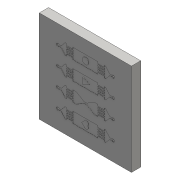
# Autodesk Inventor part: Flow-Analysis
Saved by Autodesk Inventor 2016 (Build 200138000, 138)
## iProperties
Created: 2018-10-05
Part Number: Flow-Analysis
Material: Genérico
Document SubType Name: Modeling
Designer: Joseahpacho
Density: 1 g/cm^3
Appearance: Valor por defecto
Author: Joseahpacho
Autodesk Inventor part; units mm, degrees
ref_plane "YZ Plane" through (0, 0, 0) normal (1, 0, 0) x (0, 1, 0)
ref_plane "XZ Plane" through (0, 0, 0) normal (0, 1, 0) x (-1, 0, 0)
ref_plane "XY Plane" through (0, 0, 0) normal (0, 0, 1) x (1, 0, 0)
sketch "Boceto1" plane through (0, 0, 0) normal (0, 1, 0) x (-1, 0, 0)
  line L0 (35.2407, 11.475) -> (35.2407, 10.885)
  line L1 (35.2407, 10.885) -> (31.7746, 10.885)
  line L2 (31.7746, 10.885) -> (31.7746, 11.475)
  line L3 (31.7746, 11.475) -> (35.2407, 11.475)
  line L4 (35.2407, 12.95) -> (35.2407, 12.065)
  line L5 (31.7746, 12.065) -> (31.7746, 12.95)
  line L6 (35.2407, 12.065) -> (31.7746, 12.065)
  line L7 (35.2407, 9.115) -> (35.2407, 8.525)
  line L8 (35.2407, 8.525) -> (31.7746, 8.525)
  line L9 (31.7746, 8.525) -> (31.7746, 9.115)
  line L10 (31.7746, 9.115) -> (35.2407, 9.115)
  line L11 (31.7746, 7.935) -> (35.2407, 7.935)
  line L12 (35.2407, 7.935) -> (35.2407, 7.05)
  line L13 (31.7746, 7.05) -> (31.7746, 7.935)
  line L14 (31.7746, 17.935) -> (35.2407, 17.935)
  line L15 (38.1349, 9.55) -> (36.043, 7.05)
  line L16 (35.2407, 10.295) -> (35.2407, 9.705)
  line L17 (35.2407, 9.705) -> (31.7746, 9.705)
  line L18 (31.7746, 9.705) -> (31.7746, 10.295)
  line L19 (31.7746, 10.295) -> (35.2407, 10.295)
  line L20 (31.7746, 17.05) -> (31.7746, 17.935)
  line L21 (35.2407, 17.935) -> (35.2407, 17.05)
  line L22 (35.2407, 19.115) -> (35.2407, 18.525)
  line L23 (35.2407, 18.525) -> (31.7746, 18.525)
  line L24 (31.7746, 18.525) -> (31.7746, 19.115)
  line L25 (31.7746, 19.115) -> (35.2407, 19.115)
  line L26 (18.2254, 29.705) -> (18.2254, 30.295)
  line L27 (35.2407, 31.475) -> (35.2407, 30.885)
  line L28 (38.1349, 10.45) -> (36.043, 12.95)
  line L29 (35.2407, 30.885) -> (31.7746, 30.885)
  line L30 (35.2407, 21.475) -> (35.2407, 20.885)
  line L31 (35.2407, 20.885) -> (31.7746, 20.885)
  line L32 (31.7746, 20.885) -> (31.7746, 21.475)
  line L33 (31.7746, 21.475) -> (35.2407, 21.475)
  line L34 (38.1349, 19.55) -> (36.043, 17.05)
  line L35 (31.7746, 30.885) -> (31.7746, 31.475)
  line L36 (38.1349, 20.45) -> (36.043, 22.95)
  line L37 (31.7746, 31.475) -> (35.2407, 31.475)
  line L38 (31.7746, 22.065) -> (31.7746, 22.95)
  line L39 (35.2407, 22.065) -> (31.7746, 22.065)
  line L40 (35.2407, 22.95) -> (35.2407, 22.065)
  line L41 (35.2407, 20.295) -> (35.2407, 19.705)
  line L42 (35.2407, 19.705) -> (31.7746, 19.705)
  line L43 (31.7746, 19.705) -> (31.7746, 20.295)
  line L44 (31.7746, 20.295) -> (35.2407, 20.295)
  line L45 (31.7746, 37.05) -> (31.7746, 37.935)
  line L46 (31.7746, 27.05) -> (31.7746, 27.935)
  line L47 (14.7593, 32.95) -> (14.7593, 32.065)
  line L48 (14.7593, 32.065) -> (18.2254, 32.065)
  line L49 (14.7593, 30.295) -> (14.7593, 29.705)
  line L50 (14.7593, 29.705) -> (18.2254, 29.705)
  line L51 (35.2407, 42.95) -> (35.2407, 42.065)
  line L52 (18.2254, 30.295) -> (14.7593, 30.295)
  line L53 (35.2407, 42.065) -> (31.7746, 42.065)
  line L54 (14.7593, 37.935) -> (14.7593, 37.05)
  line L55 (35.2407, 37.935) -> (35.2407, 37.05)
  line L56 (14.7593, 39.115) -> (14.7593, 38.525)
  line L57 (14.7593, 38.525) -> (18.2254, 38.525)
  line L58 (18.2254, 38.525) -> (18.2254, 39.115)
  line L59 (18.2254, 39.115) -> (14.7593, 39.115)
  line L60 (11.8651, 39.55) -> (13.957, 37.05)
  line L61 (14.7593, 40.295) -> (14.7593, 39.705)
  line L62 (14.7593, 39.705) -> (18.2254, 39.705)
  line L63 (18.2254, 39.705) -> (18.2254, 40.295)
  line L64 (18.2254, 40.295) -> (14.7593, 40.295)
  line L65 (38.1349, 29.55) -> (36.043, 27.05)
  line L66 (38.1349, 40.45) -> (36.043, 42.95)
  line L67 (11.8651, 30.45) -> (13.957, 32.95)
  line L68 (14.7593, 41.475) -> (14.7593, 40.885)
  line L69 (14.7593, 40.885) -> (18.2254, 40.885)
  line L70 (18.2254, 40.885) -> (18.2254, 41.475)
  line L71 (18.2254, 41.475) -> (14.7593, 41.475)
  line L72 (11.8651, 40.45) -> (13.957, 42.95)
  line L73 (14.7593, 42.95) -> (14.7593, 42.065)
  line L74 (18.2254, 42.065) -> (18.2254, 42.95)
  arc A0 (25.3787, 11.658) -> (23.7446, 10.0239) centre (24.5617, 10.8409) ccw
  arc A1 (23.7446, 10.0239) -> (25.3787, 8.3899) centre (24.5617, 9.2069) ccw
  line L75 (25.3787, 11.658) -> (27.0127, 10.0239)
  line L76 (27.0127, 10.0239) -> (25.3787, 8.3899)
  line L77 (25.7518, 20.4473) -> (29.9578, 22.95)
  line L78 (22.7639, 29.8706) -> (26.3406, 28.0945)
  line L79 (26.3406, 31.6467) -> (26.3406, 28.0945)
  line L80 (22.7639, 29.8706) -> (26.3406, 31.6467)
  line L81 (18.2254, 32.065) -> (18.2254, 32.95)
  line L82 (18.2254, 37.05) -> (18.2254, 37.935)
  circle A2 centre (25, 39.8706) radius 1.7363
  line L83 (18.2254, 37.935) -> (14.7593, 37.935)
  line L84 (24.2482, 20.4473) -> (25.7518, 20.4473)
  line L85 (24.2482, 20.4473) -> (20.0422, 22.95)
  line L86 (24.2482, 19.5527) -> (25.7518, 19.5527)
  line L87 (25.7518, 19.5527) -> (29.9578, 17.05)
  line L88 (24.2482, 19.5527) -> (20.0422, 17.05)
  line L89 (14.7593, 12.95) -> (14.7593, 12.065)
  line L90 (18.2254, 12.065) -> (18.2254, 12.95)
  line L91 (14.7593, 12.065) -> (18.2254, 12.065)
  line L92 (14.7593, 11.475) -> (14.7593, 10.885)
  line L93 (14.7593, 10.885) -> (18.2254, 10.885)
  line L94 (18.2254, 10.885) -> (18.2254, 11.475)
  line L95 (18.2254, 11.475) -> (14.7593, 11.475)
  line L96 (14.7593, 10.295) -> (14.7593, 9.705)
  line L97 (14.7593, 9.705) -> (18.2254, 9.705)
  line L98 (18.2254, 9.705) -> (18.2254, 10.295)
  line L99 (18.2254, 10.295) -> (14.7593, 10.295)
  line L100 (14.7593, 21.475) -> (14.7593, 20.885)
  line L101 (14.7593, 20.885) -> (18.2254, 20.885)
  line L102 (18.2254, 20.885) -> (18.2254, 21.475)
  line L103 (18.2254, 21.475) -> (14.7593, 21.475)
  line L104 (14.7593, 27.935) -> (14.7593, 27.05)
  line L105 (18.2254, 22.065) -> (18.2254, 22.95)
  line L106 (14.7593, 22.065) -> (18.2254, 22.065)
  line L107 (14.7593, 22.95) -> (14.7593, 22.065)
  line L108 (18.2254, 17.935) -> (14.7593, 17.935)
  line L109 (18.2254, 17.05) -> (18.2254, 17.935)
  line L110 (14.7593, 17.935) -> (14.7593, 17.05)
  line L111 (14.7593, 19.115) -> (14.7593, 18.525)
  line L112 (14.7593, 18.525) -> (18.2254, 18.525)
  line L113 (18.2254, 18.525) -> (18.2254, 19.115)
  line L114 (18.2254, 19.115) -> (14.7593, 19.115)
  line L115 (14.7593, 20.295) -> (14.7593, 19.705)
  line L116 (14.7593, 19.705) -> (18.2254, 19.705)
  line L117 (18.2254, 19.705) -> (18.2254, 20.295)
  line L118 (18.2254, 20.295) -> (14.7593, 20.295)
  line L119 (18.2254, 27.05) -> (18.2254, 27.935)
  line L120 (14.7593, 29.115) -> (14.7593, 28.525)
  line L121 (14.7593, 28.525) -> (18.2254, 28.525)
  line L122 (18.2254, 28.525) -> (18.2254, 29.115)
  line L123 (18.2254, 29.115) -> (14.7593, 29.115)
  line L124 (14.7593, 9.115) -> (14.7593, 8.525)
  line L125 (14.7593, 8.525) -> (18.2254, 8.525)
  line L126 (18.2254, 8.525) -> (18.2254, 9.115)
  line L127 (18.2254, 9.115) -> (14.7593, 9.115)
  line L128 (18.2254, 27.935) -> (14.7593, 27.935)
  line L129 (11.8651, 19.55) -> (13.957, 17.05)
  line L130 (11.8651, 10.45) -> (13.957, 12.95)
  line L131 (11.8651, 9.55) -> (13.957, 7.05)
  line L132 (11.8651, 29.55) -> (13.957, 27.05)
  line L133 (14.7593, 31.475) -> (14.7593, 30.885)
  line L134 (14.7593, 30.885) -> (18.2254, 30.885)
  line L135 (18.2254, 30.885) -> (18.2254, 31.475)
  line L136 (18.2254, 31.475) -> (14.7593, 31.475)
  line L137 (11.8651, 20.45) -> (13.957, 22.95)
  line L138 (31.7746, 27.935) -> (35.2407, 27.935)
  line L139 (18.2254, 7.935) -> (14.7593, 7.935)
  line L140 (14.7593, 7.935) -> (14.7593, 7.05)
  line L141 (18.2254, 7.05) -> (18.2254, 7.935)
  line L142 (35.2407, 41.475) -> (35.2407, 40.885)
  line L143 (35.2407, 40.885) -> (31.7746, 40.885)
  line L144 (31.7746, 40.885) -> (31.7746, 41.475)
  line L145 (31.7746, 41.475) -> (35.2407, 41.475)
  line L146 (31.7746, 42.065) -> (31.7746, 42.95)
  line L147 (35.2407, 27.935) -> (35.2407, 27.05)
  line L148 (31.7746, 37.935) -> (35.2407, 37.935)
  line L149 (35.2407, 39.115) -> (35.2407, 38.525)
  line L150 (35.2407, 38.525) -> (31.7746, 38.525)
  line L151 (31.7746, 38.525) -> (31.7746, 39.115)
  line L152 (31.7746, 39.115) -> (35.2407, 39.115)
  line L153 (35.2407, 40.295) -> (35.2407, 39.705)
  line L154 (35.2407, 39.705) -> (31.7746, 39.705)
  line L155 (31.7746, 39.705) -> (31.7746, 40.295)
  line L156 (31.7746, 40.295) -> (35.2407, 40.295)
  line L157 (38.1349, 30.45) -> (36.043, 32.95)
  line L158 (38.1349, 39.55) -> (36.043, 37.05)
  line L159 (31.7746, 32.065) -> (31.7746, 32.95)
  line L160 (35.2407, 32.065) -> (31.7746, 32.065)
  line L161 (35.2407, 32.95) -> (35.2407, 32.065)
  line L162 (14.7593, 42.065) -> (18.2254, 42.065)
  line L163 (35.2407, 29.115) -> (35.2407, 28.525)
  line L164 (35.2407, 28.525) -> (31.7746, 28.525)
  line L165 (31.7746, 28.525) -> (31.7746, 29.115)
  line L166 (31.7746, 29.115) -> (35.2407, 29.115)
  line L167 (35.2407, 30.295) -> (35.2407, 29.705)
  line L168 (35.2407, 29.705) -> (31.7746, 29.705)
  line L169 (31.7746, 29.705) -> (31.7746, 30.295)
  line L170 (31.7746, 30.295) -> (35.2407, 30.295)
  arc A3 (39.4, 9.55) -> (39.4, 10.45) centre (40, 10) ccw
  line L171 (38.1349, 10.45) -> (39.4, 10.45)
  line L172 (39.4, 19.55) -> (38.1349, 19.55)
  line L173 (38.1349, 20.45) -> (39.4, 20.45)
  arc A4 (39.4, 19.55) -> (39.4, 20.45) centre (40, 20) ccw
  line L174 (39.4, 9.55) -> (38.1349, 9.55)
  line L175 (10.6, 30.45) -> (11.8651, 30.45)
  arc A5 (10.6, 30.45) -> (10.6, 29.55) centre (10, 30) ccw
  line L176 (11.8651, 39.55) -> (10.6, 39.55)
  line L177 (10.6, 40.45) -> (11.8651, 40.45)
  arc A6 (10.6, 40.45) -> (10.6, 39.55) centre (10, 40) ccw
  line L178 (11.8651, 19.55) -> (10.6, 19.55)
  line L179 (10.6, 20.45) -> (11.8651, 20.45)
  arc A7 (10.6, 20.45) -> (10.6, 19.55) centre (10, 20) ccw
  arc A8 (10.6, 10.45) -> (10.6, 9.55) centre (10, 10) ccw
  line L180 (39.4, 29.55) -> (38.1349, 29.55)
  line L181 (38.1349, 30.45) -> (39.4, 30.45)
  arc A9 (39.4, 29.55) -> (39.4, 30.45) centre (40, 30) ccw
  line L182 (38.1349, 40.45) -> (39.4, 40.45)
  line L183 (39.4, 39.55) -> (38.1349, 39.55)
  line L184 (11.8651, 9.55) -> (10.6, 9.55)
  arc A10 (39.4, 39.55) -> (39.4, 40.45) centre (40, 40) ccw
  line L185 (11.8651, 29.55) -> (10.6, 29.55)
  line L186 (10.6, 10.45) -> (11.8651, 10.45)
  line L187 (50, 0) -> (50, 50)
  line L188 (50, 50) -> (0, 50)
  line L189 (0, 50) -> (0, 0)
  line L190 (0, 0) -> (50, 0)
  line L191 (14.7593, 42.95) -> (13.957, 42.95)
  line L192 (13.957, 37.05) -> (14.7593, 37.05)
  line L193 (14.7593, 32.95) -> (13.957, 32.95)
  line L194 (13.957, 27.05) -> (14.7593, 27.05)
  line L195 (36.043, 42.95) -> (35.2407, 42.95)
  line L196 (31.7746, 42.95) -> (18.2254, 42.95)
  line L197 (18.2254, 37.05) -> (31.7746, 37.05)
  line L198 (35.2407, 37.05) -> (36.043, 37.05)
  line L199 (36.043, 32.95) -> (35.2407, 32.95)
  line L200 (31.7746, 32.95) -> (18.2254, 32.95)
  line L201 (18.2254, 27.05) -> (31.7746, 27.05)
  line L202 (35.2407, 27.05) -> (36.043, 27.05)
  line L203 (36.043, 22.95) -> (35.2407, 22.95)
  line L204 (31.7746, 22.95) -> (29.9578, 22.95)
  line L205 (29.9578, 17.05) -> (31.7746, 17.05)
  line L206 (35.2407, 17.05) -> (36.043, 17.05)
  line L207 (36.043, 12.95) -> (35.2407, 12.95)
  line L208 (35.2407, 7.05) -> (36.043, 7.05)
  line L209 (13.957, 7.05) -> (14.7593, 7.05)
  line L210 (18.2254, 7.05) -> (31.7746, 7.05)
  line L211 (31.7746, 12.95) -> (18.2254, 12.95)
  line L212 (14.7593, 12.95) -> (13.957, 12.95)
  line L213 (13.957, 17.05) -> (14.7593, 17.05)
  line L214 (18.2254, 17.05) -> (20.0422, 17.05)
  line L215 (20.0422, 22.95) -> (18.2254, 22.95)
  line L216 (14.7593, 22.95) -> (13.957, 22.95)
  constraints: 434 end point, 20 point on circle, 11 centre point
sketch "Boceto2" plane through (0, 0, 0) normal (0, 1, 0) x (-1, 0, 0)
  line L0 (50, 50) -> (0, 50)
  line L1 (0, 50) -> (0, 0)
  line L2 (0, 0) -> (50, 0)
  line L3 (50, 0) -> (50, 50)
  constraints: 8 end point, 2 parallel, 1 horizontal, 1 perpendicular
extrude "Extrusión1" add sketch "Boceto2" along normal blind 5
extrude "Extrusión2" cut sketch "Boceto1" along normal blind 0.2 contours L207 L28 L171 A3 L174 L15 L208 L12 L11 L13 L210 L141 L139 L140 L209 L131 L184 A8 L186 L130 L212 L89 L91 L90 L211 L5 L6 L4 | L20 L205 L87 L86 L88 L214 L109 L108 L110 L213 L129 L178 A7 L179 L137 L216 L107 L106 L105 L215 L85 L84 L77 L204 L38 L39 L40 L203 L36 L173 A4 L172 L34 L206 L21 L14 | L197 L82 L83 L54 L192 L60 L176 A6 L177 L72 L191 L73 L162 L74 L196 L146 L53 L51 L195 L66 L182 A10 L183 L158 L198 L55 L148 L45 | L201 L119 L128 L104 L194 L132 L185 A5 L175 L67 L193 L47 L48 L81 L200 L159 L160 L161 L199 L157 L181 A9 L180 L65 L202 L147 L138 L46
sketch "Boceto3" plane through (0, 0.2, 0) normal (0, -1, 0) x (1, 0, 0)
  arc A0 (-39.4, 40.45) -> (-39.4, 39.55) centre (-40, 40) ccw projected
  arc A1 (-10.6, 39.55) -> (-10.6, 40.45) centre (-10, 40) ccw projected
  arc A2 (-10.6, 29.55) -> (-10.6, 30.45) centre (-10, 30) ccw projected
  arc A3 (-39.4, 30.45) -> (-39.4, 29.55) centre (-40, 30) ccw projected
  arc A4 (-39.4, 20.45) -> (-39.4, 19.55) centre (-40, 20) ccw projected
  arc A5 (-10.6, 19.55) -> (-10.6, 20.45) centre (-10, 20) ccw projected
  arc A6 (-10.6, 9.55) -> (-10.6, 10.45) centre (-10, 10) ccw projected
  arc A7 (-39.4, 10.45) -> (-39.4, 9.55) centre (-40, 10) ccw projected
  line L0 (-50, 0) -> (0, 0) projected
  circle A8 centre (-40, 40) radius 0.35
  circle A9 centre (-10, 40) radius 0.35
  circle A10 centre (-10, 30) radius 0.35
  circle A11 centre (-10, 20) radius 0.35
  circle A12 centre (-10, 10) radius 0.35
  circle A13 centre (-40, 10) radius 0.35
  circle A14 centre (-40, 20) radius 0.35
  circle A15 centre (-40, 30) radius 0.35
  dimension "d5" = 0.7
  dimension "d6" = 0.7
  dimension "d7" = 0.7
  dimension "d8" = 0.7
  dimension "d9" = 0.7
  dimension "d10" = 0.7
  dimension "d11" = 0.7
  dimension "d12" = 0.7
  constraints: 8 centre point, 1 coincident
  measures "d5" diameter of A8
  measures "d6" diameter of A9
  measures "d7" diameter of A10
  measures "d8" diameter of A11
  measures "d9" diameter of A12
  measures "d10" diameter of A13
  measures "d11" diameter of A14
  measures "d12" diameter of A15
extrude "Extrusión3" cut sketch "Boceto3" against normal through all
